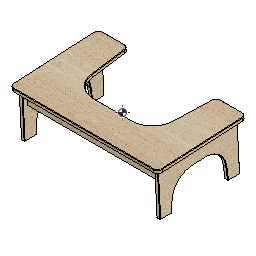
model (Autodesk Fusion 360 design; units mm, degrees)
Autodesk Fusion 360 part; units mm, degrees
sketch "top" plane through (0, 0, 0) normal (0, 0, 1) x (1, 0, 0) in component "stool"
  line L0 (0, 0) -> (500, 0)
  line L1 (120, 100.7611) -> (102.5689, 300)
  line L2 (102.5689, 300) -> (0, 300)
  line L3 (0, 300) -> (0, 0)
  line L4 (120, 100.7611) -> (380, 100.7611)
  line L5 (500, 300) -> (500, 0)
  line L6 (380, 100.7611) -> (397.4311, 300)
  line L7 (397.4311, 300) -> (500, 300)
  arc A0 (315.8568, 100.7611) -> (385.5904, 164.6602) centre (315.8568, 170.7611) ccw
  arc A1 (114.4096, 164.6602) -> (184.1432, 100.7611) centre (184.1432, 170.7611) ccw
  dimension "d5" = 300
  dimension "d6" = 500
  dimension "d7" = 260
  dimension "d8" = 200
  dimension "d21" = 70
  dimension "d36" = 95
  dimension "d37" = 95
  dimension "d42" = 294.8623
  dimension "d43" = 102.5689
  dimension "d44" = 100.7611
  constraint horizontal L0
  constraint horizontal L2
  constraint vertical L3
  constraint coincident L0.start L3.end
  constraint horizontal L4
  constraint vertical L5
  constraint horizontal L7
  constraint equal L2 L7
  constraint equal L3 L5
  constraint tangent L4 A0
  constraint coincident L4 A0.start
  constraint coincident L6 A0.end
  constraint tangent L1 A1
  constraint coincident L1 A1.start
  constraint coincident L4 A1.end
  constraint tangent L6 A0
  constraint tangent L4 A1
  constraint equal A0 A1
  measures "d5" distance of L0.start L2.end
  measures "d6" distance of L0.start L0.end
  measures "d7" distance of L1.start L4.end
  measures "d8" distance of L1.end L1.start
  measures "d21" radius of A0
  measures "d36" angle of L6 L7
  measures "d37" angle of L1 L2
  measures "d42" distance of L1.end L6.end
  measures "d43" distance of L6.end L5.start
  measures "d44" vertical distance of L0.end L4.end
extrude "Extrude1" add sketch "top" along normal blind 12 makes body 1 in component "stool"
move_body "Move1" bodies 1 to x (1, 0, 0) y (0, 0.99863, 0.052336) z (0, -0.052336, 0.99863) at (0, 1.8303, 0.0799) in component "stool"
sketch "side" plane through (0, 0, 0) normal (1, 0, 0) x (0, 1, 0) in component "stool"
  line L0 (285.4411, 14.9433) -> (294.0373, -149.0827)
  line L1 (294.0373, -149.0827) -> (254.0373, -149.0827)
  line L2 (254.0373, -149.0827) -> (247.5748, -103.0993)
  arc A0 (247.5748, -103.0993) -> (174.5925, -42.9374) centre (178.256, -112.8414) ccw
  line L3 (174.5925, -42.9374) -> (133.2386, -45.1046)
  arc A1 (133.2386, -45.1046) -> (66.9447, -112.5657) centre (136.9021, -115.0087) ccw
  line L4 (66.9447, -112.5657) -> (65.6695, -149.0827)
  line L5 (65.6695, -149.0827) -> (25.6695, -149.0827)
  line L6 (25.6695, -149.0827) -> (17.8083, 0.9173)
  line L7 (285.4411, 14.9433) -> (17.8083, 0.9173)
  line L8 (301.4191, 15.7807) -> (1.8303, 0.0799)
  line L9 (285.4411, 14.9433) -> (285.2317, 18.9378)
  line L10 (285.2317, 18.9378) -> (17.599, 4.9118)
  line L11 (17.599, 4.9118) -> (17.8083, 0.9173)
  dimension "d15" = 40
  dimension "d18" = 70
  dimension "d45" = 5
  dimension "d46" = 5
  dimension "d47" = 16
  dimension "d48" = 16
  dimension "d49" = 150
  dimension "d50" = 52
  dimension "d58" = 4
  constraint tangent L2 A0
  constraint tangent A0 L3
  constraint tangent L3 A1
  constraint tangent A1 L4
  constraint horizontal L5
  constraint equal L1 L5
  constraint equal A0 A1
  constraint perpendicular L6 L7
  constraint horizontal L1
  constraint perpendicular L0 L7
  constraint coincident L6.end L8
  constraint coincident L0.start L8
  constraint collinear L1 L5
  constraint parallel L3 L7
  constraint collinear L0 L9
  constraint collinear L6 L11
  constraint parallel L7 L10
  measures "d15" distance of L0.end L1.end
  measures "d18" radius of A0
  measures "d45" angle of L0 L2
  measures "d46" angle of L4 L6
  measures "d47" distance of L0.start L8.start
  measures "d48" distance of L6.end L8.end
  measures "d49" vertical distance of L5.end L6.end
  measures "d50" distance of L3 L7
  measures "d58" distance of L6.end L10.end
extrude "Extrude2" add sketch "side" along normal blind 12 from surface at 16 separate body makes body 2 in component "stool"
ref_plane "WorkPlane1" through (250, 151.3107, 13.9221) normal (-1, 0, 0) x (0, -0.99863, -0.052336) in component "stool"
mirror "Mirror1" about plane through (250, 151.3107, 13.9221) normal (-1, 0, 0) of bodies 2 makes body 3 in component "stool"
sketch "stretcher" plane through (28, 0, 0) normal (1, 0, 0) x (0, 1, 0) in component "stool"
  line L0 (294.0373, -149.0827) -> (285.2317, 18.9378)
  line L1 (17.599, 4.9118) -> (25.6695, -149.0827)
  line L2 (25.6695, -149.0827) -> (65.6695, -149.0827)
  line L3 (65.6695, -149.0827) -> (66.9447, -112.5657)
  arc A0 (133.2386, -45.1046) -> (66.9447, -112.5657) centre (136.9021, -115.0087) ccw
  line L4 (133.2386, -45.1046) -> (174.5925, -42.9374)
  arc A1 (247.5748, -103.0993) -> (174.5925, -42.9374) centre (178.256, -112.8414) ccw
  line L5 (247.5748, -103.0993) -> (254.0373, -149.0827)
  line L6 (254.0373, -149.0827) -> (294.0373, -149.0827)
  line L7 (285.4411, 14.9433) -> (17.8083, 0.9173)
  line L8 (33.7864, 1.7547) -> (36.5079, -50.1741)
  line L9 (36.5079, -50.1741) -> (48.4914, -49.546)
  line L10 (48.4914, -49.546) -> (45.77, 2.3827)
  line L11 (285.2317, 18.9378) -> (17.599, 4.9118)
  line L12 (45.77, 2.3827) -> (45.5606, 6.3772)
  line L13 (33.7864, 1.7547) -> (33.5771, 5.7492)
  dimension "d51" = 12
  dimension "d52" = 16
  dimension "d53" = 52
  constraint parallel L8 L10
  constraint equal L8 L10
  constraint coincident L11 L12.end
  constraint perpendicular L11 L12
  constraint coincident L11 L13.end
  constraint perpendicular L11 L13
  measures "d51" distance of L8.end L9.end
  measures "d52" distance of L7.end L8.start
  measures "d53" distance of L8.start L8.end
extrude "Extrude4" add sketch "stretcher" along normal up to surface (452 mm away) from surface at -4 separate body contours L7 L8 L9 L10 | L7 L11 L12 L13 makes body 4 in component "stool"
combine "Combine1" operation cut target body 1 tool bodies 2 4 3 keep tools in component "stool"
combine "Combine2" operation cut target body 2 tool bodies 4 keep tools in component "stool"
combine "Combine3" operation cut target body 3 tool bodies 4 keep tools in component "stool"
fillet "Fillet1" radius 16 6 edges at (0, 301.1051, 21.7725) (0, 1.5163, 6.0717) (500, 1.5163, 6.0717) (500, 301.1051, 21.7725) (102.5689, 301.1051, 21.7725) (397.4311, 301.1051, 21.7725) on bodies 1 in component "stool"
fillet "Fillet2" radius 1.5875 46 edges at (495.3137, 6.5101, 0.3252) (250, 1.8303, 0.0799) (4.6863, 6.5101, 0.3252) (0, 151.6247, 7.9303) (4.6863, 296.7393, 15.5354) (51.9538, 301.4191, 15.7807) (98.717, 297.2213, 15.5607) (109.1281, 226.5492, 11.8569) (136.8519, 120.8186, 6.3158) (250, 102.4532, 5.3533) (363.1481, 120.8186, 6.3158) (390.8719, 226.5492, 11.8569) (401.283, 297.2213, 15.5607) (448.0462, 301.4191, 15.7807) (495.3137, 296.7393, 15.5354) (500, 151.6247, 7.9303) (16, 250.806, -126.091) (16, 222.7815, -58.8277) (16, 153.9155, -44.021) (16, 86.9745, -65.9451) (16, 66.3071, -130.8242) (16, 21.6343, -72.0855) (28, 21.6343, -72.0855) (28, 289.6345, -65.0724) (16, 289.6345, -65.0724) (28, 66.3071, -130.8242) (28, 86.9745, -65.9451) (28, 153.9155, -44.021) (28, 222.7815, -58.8277) (28, 250.806, -126.091) (472, 66.3071, -130.8242) (472, 86.9745, -65.9451) (472, 153.9155, -44.021) (472, 222.7815, -58.8277) (472, 250.806, -126.091) (484, 250.806, -126.091) (484, 222.7815, -58.8277) (484, 153.9155, -44.021) (484, 86.9745, -65.9451) (484, 66.3071, -130.8242) (472, 21.6343, -72.0855) (484, 21.6343, -72.0855) (484, 289.6345, -65.0724) (472, 289.6345, -65.0724) (250, 36.5079, -50.1741) (250, 48.4914, -49.546) 5 faces at (461.8635, 155.8767, 20.1696) (20, 280.704, -149.0827) (20, 52.3362, -149.0827) (476, 280.704, -149.0827) (480, 52.3362, -149.0827) on bodies 1 2 3 4 in component "stool"
component "stool" placed x (1, 0, 0) y (0, 1, 0) z (0, 0, 1) at (0, 0, 0)
equation "width = 500 mm"
equation "depth = 300 mm"
equation "holeWidth = 260 mm"
equation "holeDepth = 200 mm"
equation "d5 = depth"
equation "d6 = width"
equation "d7 = holeWidth"
equation "d8 = holeDepth"
equation "thickness = 12 mm"
equation "d10 = thickness"
equation "inset = 16 mm"
equation "d15 = memberWidth"
equation "height = 150 mm"
equation "d18 = largeRadius"
equation "memberWidth = 40 mm"
equation "largeRadius = 70 mm"
equation "d21 = largeRadius"
equation "d22 = inset"
equation "d23 = thickness"
equation "stretcherWidth = memberWidth * 1.3"
equation "taper = 5 deg"
equation "d36 = 90 deg + taper"
equation "d37 = 90 deg + taper"
equation "d39 = inset"
equation "d41 = finishRoundover"
equation "d45 = taper"
equation "d46 = taper"
equation "d47 = inset"
equation "d48 = inset"
equation "d49 = height"
equation "d50 = stretcherWidth"
equation "d51 = thickness"
equation "d52 = inset"
equation "d53 = stretcherWidth"
equation "d54 = -dadoDepth"
equation "finishRoundover = 1/16\""
equation "dadoDepth = thickness / 3"
equation "d58 = dadoDepth"
equation "d59 = -dadoDepth"
named bodies: "top", "lhs leg", "rhs leg", "stretcher"
